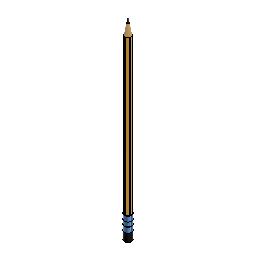
N2 Pencil v1 (Autodesk Fusion 360 design; units mm, degrees)
Autodesk Fusion 360 part; units mm, degrees
sketch "Sketch1" plane through (0, 0, 0) normal (0, 0, 1) x (1, 0, 0)
  line L0 (-1.27, 1.748) -> (-2.0549, -0.6677)
  line L1 (-2.0549, -0.6677) -> (0, -2.1607)
  line L2 (0, -2.1607) -> (2.0549, -0.6677)
  line L3 (2.0549, -0.6677) -> (1.27, 1.748)
  line L4 (1.27, 1.748) -> (-1.27, 1.748)
  line L5 (0, 0) -> (0, 1.748) construction
  line L6 (0, 0) -> (-12.7, 0) construction
  dimension "d1" = 2.54
  dimension "d2" = 12.7
  dimension "d3" = 90
  constraint coincident L5.start L6.start
  constraint midpoint L4 L5.end
  constraint horizontal L6
  measures "d1" distance of L0.start L3.end
  measures "d2" distance of L5.start L6.end
  measures "d3" angle of L5 L6
extrude "Extrude1" add sketch "Sketch1" along normal blind 88.9 makes body 1
sketch "Sketch2" plane through (0, 0, 0) normal (0, 0, -1) x (1, 0, 0)
  line L0 (-1.27, -1.748) -> (1.27, -1.748)
  line L1 (1.27, -1.748) -> (2.0549, 0.6677)
  line L2 (2.0549, 0.6677) -> (0, 2.1607)
  line L3 (0, 2.1607) -> (-2.0549, 0.6677)
  line L4 (-2.0549, 0.6677) -> (-1.27, -1.748)
  circle A0 centre (0, 0) radius 2.1607
  constraint coincident A0.centre origin
  constraint coincident L0.start A0
extrude "Extrude2" add sketch "Sketch2" along normal blind 3.048 bodies 1
sketch "Sketch3" plane through (0, 0, -3.048) normal (0, 0, -1) x (1, 0, 0)
  circle A0 centre (0, 0) radius 2.1607
  circle A1 centre (0, 0) radius 2.0845
  dimension "d8" = -0.0762
extrude "Extrude3" add sketch "Sketch3" along normal blind 2.54 contours A1 bodies 1
sketch "Sketch4" plane through (0, 0, -5.588) normal (0, 0, -1) x (1, 0, 0)
  circle A0 centre (0, 0) radius 2.0845
  circle A1 centre (0, 0) radius 2.1607
extrude "Extrude4" add sketch "Sketch4" along normal blind 3.048 contours A0 | A1 bodies 1
sketch "Sketch5" plane through (0, 0, -8.636) normal (0, 0, -1) x (1, 0, 0)
  circle A0 centre (0, 0) radius 2.1607
  circle A1 centre (0, 0) radius 2.1099
  dimension "d14" = 0.0508
  constraint coincident A0.centre A1.centre
  measures "d14" distance of A0 A1
extrude "Extrude5" add sketch "Sketch5" along normal blind 5.08 contours A1 bodies 1
fillet "Fillet1" radius 0.508 1 edges at (-1.9671, 0.763, -13.716) on bodies 1
chamfer "Chamfer1" distance 0.0508 angle 45 2 edges at (-1.9434, -0.7538, -3.048) (-1.9434, 0.7538, -5.588) on bodies 1
fillet "Fillet2" radius 0.127 5 edges at (0, 2.1607, 0) (-2.0549, 0.6677, 0) (2.0549, 0.6677, 0) (-1.27, -1.748, 0) (1.27, -1.748, 0) on bodies 1
fillet "Fillet3" radius 0.635 5 edges at (-2.0549, -0.6677, 44.3865) (0, -2.1607, 44.3865) (2.0549, -0.6677, 44.3865) (-1.27, 1.748, 44.3865) (1.27, 1.748, 44.3865) on bodies 1
sketch "Sketch7" plane through (0, 0, 88.9) normal (0, 0, 1) x (-1, 0, 0)
  arc A0 (-1.4126, -1.3092) -> (-0.8086, -1.748) centre (-0.8086, -1.113) ccw
  line L0 (-0.8086, -1.748) -> (0.8086, -1.748)
  arc A1 (0.8086, -1.748) -> (1.4126, -1.3092) centre (0.8086, -1.113) ccw
  line L1 (1.4126, -1.3092) -> (1.9123, 0.2289)
  arc A2 (1.9123, 0.2289) -> (1.6817, 0.9389) centre (1.3084, 0.4251) ccw
  line L2 (1.6817, 0.9389) -> (0.3732, 1.8895)
  arc A3 (0.3732, 1.8895) -> (-0.3732, 1.8895) centre (0, 1.3757) ccw
  line L3 (-0.3732, 1.8895) -> (-1.6817, 0.9389)
  arc A4 (-1.6817, 0.9389) -> (-1.9123, 0.2289) centre (-1.3084, 0.4251) ccw
  line L4 (-1.9123, 0.2289) -> (-1.4126, -1.3092)
  circle A5 centre (0, 0) radius 1.748
  constraint coincident A5.centre origin
  constraint tangent L0 A5
extrude "Extrude6" add sketch "Sketch7" along normal blind 6.35 draft -10 contours A5 bodies 1
sketch "Sketch8" plane through (0, 0, 95.25) normal (0, 0, 1) x (-1, 0, 0)
  circle A0 centre (0, 0) radius 0.6283
  circle A1 centre (0, 0) radius 0.6283
  constraint coincident A0.centre A1.centre
  constraint equal A0 A1
extrude "Extrude7" add sketch "Sketch8" along normal blind 3.81 draft -10 separate body makes body 2
sketch "Sketch9" plane through (-1.6625, 0.5402, 0) normal (-0.951057, 0.309017, 0) x (-0.309017, -0.951057, 0)
  line L0 (-0.8086, 88.9) -> (-0.8086, 0)
  line L1 (-0.8086, 0) -> (0.8086, 0)
  line L2 (0.8086, 0) -> (0.8086, 88.9)
  line L3 (0.8086, 88.9) -> (0, 88.9)
  line L4 (0, 88.9) -> (-0.8086, 88.9)
  dimension "d28" = 1.27
  text T0 "How to CAD Almost Anything!" font "Arial" height 1.27 align centre spacing 1 along the path L0 letters at x, y, angle (0.7975, 56.2408, -90) (0.7975, 54.9596, -90) (0.7975, 53.9728, -90) (0.7975, 52.6916, -90) (0.7975, 52.1986, -90) (0.7975, 51.7057, -90) (0.7975, 50.719, -90) (0.7975, 50.2261, -90) (0.7975, 48.9448, -90) (0.7975, 47.7562, -90) (0.7975, 46.475, -90) (0.7975, 45.9821, -90) (0.7975, 44.7935, -90) (0.7975, 44.3993, -90) (0.7975, 42.9214, -90) (0.7975, 41.9347, -90) (0.7975, 41.0476, -90) (0.7975, 40.5547, -90) (0.7975, 40.0617, -90) (0.7975, 38.8732, -90) (0.7975, 37.8865, -90) (0.7975, 36.9994, -90) (0.7975, 36.5064, -90) (0.7975, 35.5197, -90) (0.7975, 35.1255, -90) (0.7975, 34.1388, -90) (0.7975, 33.1521, -90)
extrude "Extrude8" cut sketch "Sketch9" against normal blind 0.254 text T0 bodies 1
